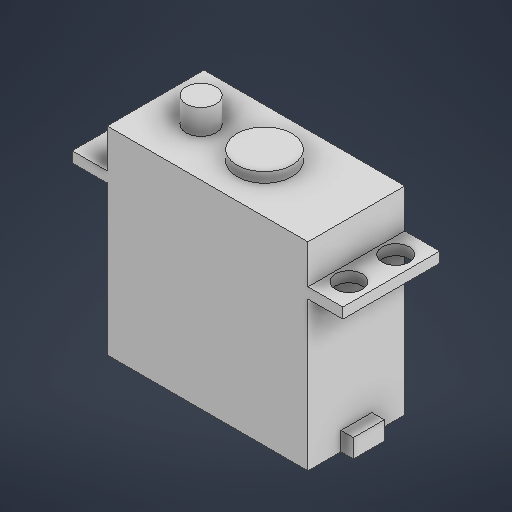
# Autodesk Inventor part: Servo
Saved by Autodesk Inventor 2026.2 (Build 302298000, 298)
## iProperties
Created: 2026-02-24
Part Number: Servo
Material: Generic
Document SubType Name: Modeling
Designer: chigg
Density: 1 g/cm^3
Appearance: Default
Author: chigg
Autodesk Inventor part; units mm, degrees
ref_plane "YZ Plane" through (0, 0, 0) normal (1, 0, 0) x (0, 1, 0)
ref_plane "XZ Plane" through (0, 0, 0) normal (0, 1, 0) x (-1, 0, 0)
ref_plane "XY Plane" through (0, 0, 0) normal (0, 0, 1) x (1, 0, 0)
sketch "Sketch1" plane through (0, 0, 0) normal (0, 1, 0) x (-1, 0, 0)
  line L0 (13.3986, -11.7687) -> (-26.8014, -11.7687)
  line L1 (-26.8014, -11.7687) -> (-26.8014, 7.6313)
  line L2 (-26.8014, 7.6313) -> (13.3986, 7.6313)
  line L3 (13.3986, 7.6313) -> (13.3986, -11.7687)
  point P0 (0, 0)
  dimension "d0" = 19.4
  dimension "d1" = 40.2
  constraints: 8 end point, 2 parallel, 1 horizontal, 1 perpendicular
  measures "d0" distance of L0.end L1.end
  measures "d1" distance of L0.start L0.end
extrude "Extrusion1" add sketch "Sketch1" along normal blind 39.7
sketch "Sketch2" plane through (26.8014, 0, 7.6313) normal (1, 0, 0) x (0, 0, -1)
  line L0 (6.6, 3.7) -> (12.8, 3.7)
  line L1 (12.8, 3.7) -> (12.8, 0)
  line L2 (12.8, 0) -> (6.6, 0)
  line L3 (6.6, 0) -> (6.6, 3.7)
  line L4 (19.4, 0) -> (19.4, 39.7) projected
  line L5 (0, 0) -> (0, 39.7) projected
  line L6 (0, 0) -> (19.4, 0) projected
  point P0 (7.6313, 0)
  point P1 (12.8, 1.85)
  point P2 (6.6, 1.85)
  dimension "d4" = 6.2
  dimension "d5" = 3.7
  dimension "d6" = 6.6
  dimension "d7" = 6.6
  dimension "d8" = 0
  constraints: 8 end point, 2 midpoint, 2 parallel, 1 horizontal, 1 perpendicular
  measures "d4" distance of L0.start L0.end
  measures "d5" distance of L0.end L1.end
  measures "d6" distance from line of L4 point (12.8, 1.85)
  measures "d7" distance from line of point (6.6, 1.85) L5
  measures "d8" distance between parallel lines of L6 L2
extrude "Extrusion2" add sketch "Sketch2" along normal blind 2.5
sketch "Sketch5" plane through (-13.3986, 0, -11.7687) normal (-1, 0, 0) x (0, 0, 1)
  line L0 (6.6, 3.7) -> (12.8, 3.7) projected
  line L1 (6.6, 3.7) -> (12.8, 3.7)
  line L2 (12.8, 3.7) -> (12.8, 0)
  line L3 (12.8, 0) -> (6.6, 0)
  line L4 (6.6, 0) -> (6.6, 3.7)
  point P0 (11.7687, 0)
  constraints: 8 end point, 3 perpendicular, 1 collinear
extrude "Extrusion3" add sketch "Sketch5" along normal blind 2.5
sketch "Sketch6" plane through (26.8014, 0, -11.7687) normal (1, 0, 0) x (0, 0, -1)
  line L0 (-19.4, 0) -> (-19.4, 39.7) projected
  line L1 (0, 0) -> (0, 39.7) projected
  line L2 (-19.4, 31.9) -> (0, 31.9)
  line L3 (0, 31.9) -> (0, 29.8)
  line L4 (0, 29.8) -> (-19.4, 29.8)
  line L5 (-19.4, 29.8) -> (-19.4, 31.9)
  line L6 (-19.4, 39.7) -> (0, 39.7) projected
  point P0 (-11.7687, 0)
  point P1 (0, 31.9)
  dimension "d13" = 2.1
  dimension "d14" = 7.8
  constraints: 8 end point, 2 parallel, 2 point on line, 1 horizontal, 1 perpendicular
  measures "d13" distance between parallel lines of L4 L2
  measures "d14" distance between parallel lines of L6 L2
extrude "Extrusion4" add sketch "Sketch6" along normal blind 7 contours L0 L2 L1 L4
sketch "Sketch7" plane through (-13.3986, 0, 7.6313) normal (-1, 0, 0) x (0, 0, 1)
  line L0 (-19.4, 29.8) -> (-19.4, 31.9) projected
  line L1 (-19.4, 29.8) -> (-19.4, 31.9)
  line L2 (0, 31.9) -> (0, 29.8) projected
  line L3 (-19.4, 31.9) -> (0, 31.9)
  line L4 (0, 31.9) -> (0, 29.8)
  line L5 (0, 29.8) -> (-19.4, 29.8)
  point P0 (-7.6313, 0)
  constraints: 8 end point, 2 collinear, 2 perpendicular
extrude "Extrusion5" add sketch "Sketch7" along normal blind 7
sketch "Sketch8" plane through (0, 39.7, 0) normal (0, 1, 0) x (1, 0, 0)
  circle A0 centre (8.4014, 2.0687) radius 5.5
  line L0 (26.8014, -7.6313) -> (26.8014, 11.7687) projected
  line L1 (26.8014, 11.7687) -> (-13.3986, 11.7687) projected
  point P0 (0, 0)
  dimension "d19" = 11
  dimension "d20" = 18.4
  dimension "d23" = 9.7
  constraints: 1 centre point
  measures "d19" diameter of A0
  measures "d20" distance from line of L0 A0.centre
  measures "d23" distance from line of L1 A0.centre
extrude "Extrusion6" add sketch "Sketch8" along normal blind 2
sketch "Sketch10" plane through (0, 39.7, 0) normal (0, 1, 0) x (1, 0, 0)
  circle A0 centre (-4.2986, 2.0687) radius 3
  line L0 (-13.3986, 11.7687) -> (-13.3986, -7.6313) projected
  point P0 (0, 0)
  dimension "d26" = 6
  dimension "d27" = 9.1
  constraints: 1 centre point
  measures "d26" diameter of A0
  measures "d27" distance from line of L0 A0.centre
extrude "Extrusion7" add sketch "Sketch10" along normal blind 5
sketch "Sketch11" plane through (26.8014, 31.9, 7.6313) normal (0, 1, 0) x (1, 0, 0)
  circle A0 centre (3.2, 5) radius 2.7
  line L0 (0, 0) -> (7, 0) projected
  circle A1 centre (3.2, 14.4) radius 2.7
  line L1 (0, 19.4) -> (7, 19.4) projected
  line L2 (0, 0) -> (0, 19.4) projected
  line L3 (7, 19.4) -> (7, 0) projected
  point P0 (-26.8014, 7.6313)
  dimension "d30" = 5.4
  dimension "d31" = 5
  dimension "d32" = 5
  dimension "d33" = 5.4
  dimension "d38" = 3.8
  dimension "d39" = 3.8
  constraints: 2 centre point
  measures "d30" diameter of A0
  measures "d31" distance from line of L0 A0.centre
  measures "d32" distance from line of L1 A1.centre
  measures "d33" diameter of A1
  measures "d38" distance from line of L3 A0.centre
  measures "d39" distance from line of L3 A1.centre
extrude "Extrusion8" cut sketch "Sketch11" against normal blind 5 contours A0 | A1
equation "\"d31\" = d32"
equation "\"d33\" = d30"
equation "\"d39\" = d38"
body "Solid1"
